End covers (Autodesk Fusion 360 design; units mm, degrees)
Autodesk Fusion 360 part; units mm, degrees
sketch "Sketch1" plane through (0, 0, 0) normal (0, 0, 1) x (1, 0, 0)
  line L0 (0, 0) -> (42.05, 0)
  line L1 (42.05, 0) -> (42.05, 42)
  line L2 (42.05, 42) -> (0, 42)
  line L3 (0, 42) -> (0, 0)
  line L4 (0, 42) -> (12, 42)
  circle A0 centre (0, 42) radius 12
  circle A1 centre (42.05, 42) radius 12
  circle A2 centre (0, -0.05) radius 12
  circle A3 centre (42.05, -0.05) radius 12
  line L5 (41.025, 46) -> (1.025, 46)
  line L6 (-3.975, 41) -> (-3.975, 1)
  line L7 (1.025, -4) -> (41.025, -4)
  line L8 (46.025, 1) -> (46.025, 41)
  line L9 (46.025, 46) -> (-3.975, -4) construction
  line L10 (-3.975, 46) -> (46.025, -4) construction
  arc A4 (1.025, 46) -> (-3.975, 41) centre (1.025, 41) ccw
  arc A5 (46.025, 41) -> (41.025, 46) centre (41.025, 41) ccw
  arc A6 (41.025, -4) -> (46.025, 1) centre (41.025, 1) ccw
  arc A7 (-3.975, 1) -> (1.025, -4) centre (1.025, 1) ccw
  line L11 (0, 1.4491) -> (1.4491, 0)
  line L12 (40.5759, -0.025) -> (42.025, 1.4241)
  line L13 (42.05, 40.5509) -> (40.6009, 42)
  line L14 (1.4741, 42.025) -> (0.025, 40.5759)
  point P0 (21.025, 21)
  point P1 (21.025, 21)
  dimension "d1" = 42
  dimension "d2" = 42.05
  dimension "d3" = 12
  dimension "d6" = 42.05
  dimension "d7" = -42.05
  dimension "d10" = 21
  dimension "d11" = 21.025
  dimension "d12" = 50
  dimension "d13" = 50
  dimension "d14" = 5
  dimension "d21" = 1.45
  dimension "d23" = 360
  constraint horizontal L0
  constraint vertical L1
  constraint horizontal L2
  constraint vertical L3
  constraint coincident L0.start L3.end
  constraint perpendicular L3 L4
  constraint coincident L2.end L3.start
  constraint coincident L4.end A0
  constraint horizontal L5
  constraint perpendicular L5 L6
  constraint parallel L5 L7
  constraint parallel L6 L8
  constraint coincident L9 P1
  constraint coincident L10 P1
  constraint coincident P1 P0
  constraint coincident L10.start L6
  constraint coincident L10.start L5
  constraint tangent L6 A4
  constraint tangent L5 A4
  constraint coincident L9.start L8
  constraint coincident L9.start L5
  constraint tangent L8 A5
  constraint tangent L5 A5
  constraint equal A4 A5
  constraint coincident L10.end L7
  constraint coincident L10.end L8
  constraint tangent L7 A6
  constraint tangent L8 A6
  constraint equal A4 A6
  constraint coincident L9.end L7
  constraint coincident L9.end L6
  constraint tangent L7 A7
  constraint tangent L6 A7
  constraint equal A4 A7
  constraint coincident L3 L11.start
  constraint coincident L0 L11.end
  constraint perpendicular L9 L11
  measures "d1" distance of L0.start L2.end
  measures "d2" distance of L0.start L0.end
  measures "d3" distance of L2.end L4.end
  measures "d10" distance of L2 P1
  measures "d11" distance of L3 P1
  measures "d12" distance of L10.start L9.end
  measures "d13" distance of L9.end L10.end
  measures "d14" radius of A4
  measures "d21" distance of A2.centre L11.end
extrude "Extrude2" add sketch "Sketch1" along normal blind 3 contours L0 L3 L11 | L0 L3 A2 L6 L7 A7 | L0 L3 A2 L11 | L0 L1 L2 L3 A0 A1 A2 A3 | L0 A2 A3 L7 | L3 A0 A2 L6 | L0 L1 A3 | L0 L1 A3 L7 L8 A6 | L2 L3 L4 A0 L5 L6 A4 | L2 L3 L4 A0 | L1 A1 A3 L8 | L2 A0 A1 L5 | L1 L2 A1 L13 | L1 L2 A1 L5 L8 A5 | L1 L2 L13
extrude "Extrude3" add sketch "Sketch1" against normal blind 3 contours L0 L3 L11 | L0 L3 A2 L11 | L0 L1 A3 | L2 L3 L4 A0 | L1 L2 A1 L13 | L1 L2 L13
fillet "Fillet1" radius 3 8 edges at (44.5605, -2.5355, 3) (46.025, 21, 3) (44.5605, 44.5355, 3) (21.025, 46, 3) (-2.5105, 44.5355, 3) (-3.975, 21, 3) (-2.5105, -2.5355, 3) (21.025, -4, 3)
extrude "Extrude5" cut sketch "Sketch1" along normal blind 1.5 contours L0 L1 L2 L3 A0 A1 A2 A3
